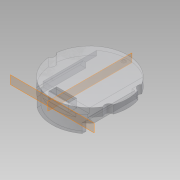
# Autodesk Inventor part: bottom2_2
Saved by Autodesk Inventor 2015 SP2 (Build 190223200, 223)
## iProperties
Created: 2015-01-05
Part Number: bottom2_2
Material: Acrylic
Document SubType Name: Modeling
Designer: Mathieu
Density: 1.188 g/cm^3
Appearance: Transparent - Clear
Mass: 1.09009 g
Surface Area: 15.2102 cm^2
Volume: 0.917582 cm^3
Author: Mathieu
Autodesk Inventor part; units mm, degrees
ref_plane "YZ Plane" through (0, 0, 0) normal (1, 0, 0) x (0, 1, 0)
ref_plane "XZ Plane" through (0, 0, 0) normal (0, 1, 0) x (-1, 0, 0)
ref_plane "XY Plane" through (0, 0, 0) normal (0, 0, 1) x (1, 0, 0)
sketch "Sketch10" plane through (0, 0, 0) normal (0, 1, 0) x (-1, 0, 0)
  circle A0 centre (0, 0) radius 12.25
  dimension "d115" = 24.5
  constraints: 1 centre point
  measures "d115" diameter of A0
extrude "Extrusion8" add sketch "Sketch10" along normal blind 2.7
sketch "Sketch15" plane through (0, 0, 0) normal (0, -1, 0) x (1, 0, 0)
  circle A0 centre (0, 0) radius 12.75 construction
  line L0 (12.75, 0) -> (0, 0) construction
  line L1 (0, 0) -> (-11.5554, -5.3884) construction
  line L2 (0, 0) -> (-11.5554, 5.3884) construction
  circle A1 centre (-11.5554, -5.3884) radius 1.375
  circle A2 centre (12.75, 0) radius 1.375
  circle A3 centre (-11.5554, 5.3884) radius 1.375
  dimension "d116" = 25.5
  dimension "d117" = 25
  dimension "d118" = 25
  dimension "d119" = 2.75
  constraints: 6 end point, 4 centre point, 4 coincident, 3 point on circle, 2 equal radius, 1 horizontal
  measures "d116" diameter of A0
  measures "d117" angle of L2 L0
  measures "d118" angle of L1 L0
  measures "d119" diameter of A2
extrude "Extrusion13" cut sketch "Sketch15" against normal up to surface (2.7 mm away)
sketch "Sketch17" plane through (0, 2.7, 0) normal (0, 1, 0) x (1, 0, 0)
  line L0 (-3.885, 10.76) -> (2.615, 10.76)
  line L1 (2.615, 10.76) -> (2.615, 8.16)
  line L2 (2.615, 8.16) -> (-3.885, 8.16)
  line L3 (-3.885, 8.16) -> (-3.885, 10.76)
  line L4 (2.615, 8.16) -> (-3.885, 10.76) construction
  line L5 (-3.885, 8.16) -> (2.615, 10.76) construction
  point P0 (0, 0)
  point P1 (-0.635, 9.46)
  dimension "d130" = 2.6
  dimension "d131" = 6.5
  dimension "d144" = 9.46
  dimension "d145" = 0.635
  constraints: 12 end point, 2 midpoint, 2 parallel, 1 horizontal, 1 perpendicular
  measures "d130" distance of L2.end L0.start
  measures "d131" distance of L1.end L2.end
  measures "d144" vertical distance of point (0, 0) point (-0.635, 9.46)
  measures "d145" horizontal distance of point (0, 0) point (-0.635, 9.46)
extrude "Extrusion14" cut sketch "Sketch17" against normal up to next
sketch "Sketch11" plane through (0, 0, 0) normal (0, -1, 0) x (1, 0, 0)
  line L0 (7.5, -7.7326) -> (-7.5, -7.7326)
  line L1 (-7.5, -7.7326) -> (-7.5, 12.25)
  line L2 (-7.5, 12.25) -> (7.5, 12.25)
  line L3 (7.5, 12.25) -> (7.5, -7.7326)
  arc A0 (12.1857, 1.2539) -> (12.1857, -1.2539) centre (12.75, 0) ccw projected
  arc A1 (-10.5141, -6.2863) -> (12.1857, -1.2539) centre (0, 0) ccw projected
  arc A2 (-10.5141, -6.2863) -> (-11.5739, -4.0135) centre (-11.5554, -5.3884) ccw projected
  arc A3 (-11.5739, 4.0135) -> (-11.5739, -4.0135) centre (0, 0) ccw projected
  arc A4 (-11.5739, 4.0135) -> (-10.5141, 6.2863) centre (-11.5554, 5.3884) ccw projected
  arc A5 (12.1857, 1.2539) -> (-10.5141, 6.2863) centre (0, 0) ccw projected
  dimension "d78" = 15
  dimension "d122" = 7.5
  constraints: 8 end point, 2 parallel, 1 horizontal, 1 perpendicular, 1 tangent
  measures "d78" distance of L0.start L0.end
  measures "d122" distance from line of point (0, 0) L3
extrude "Extrusion9" cut sketch "Sketch11" against normal blind 1.54 contours L0 L1 A5 L3 | A5 L2 L3 | L1 L2 A5
ref_plane "Work Plane4" through (0, 0, -12.25) normal (0, 0, -1) x (-1, 0, 0)
ref_plane "Work Plane3" through (0, 0, -7.7326) normal (-1, 0, 0) x (0, 0, 1)
sketch "Sketch13" plane through (0, 0, -12.25) normal (0, 0, -1) x (-1, 0, 0)
  line L0 (-7.5, 1.54) -> (-7.5, 0) projected
  line L1 (-12.1857, 0) -> (-7.5, 0) projected
  line L2 (-12.1857, 0) -> (-12.1857, 2.7) projected
  line L3 (10.5141, 2.7) -> (-12.1857, 2.7) projected
  line L4 (10.5141, 2.7) -> (10.5141, 0) projected
  line L5 (7.5, 0) -> (10.5141, 0) projected
  line L6 (7.5, 0) -> (7.5, 1.54) projected
  line L7 (7.5, 1.54) -> (-7.5, 1.54) projected
  line L8 (7.5, 0) -> (7.5, -1.6588)
  line L9 (7.5, -1.6588) -> (9.3, -1.6588)
  line L10 (9.3, -1.6588) -> (8.4, -0.1)
  line L11 (8.4, -0.1) -> (8.4, 0)
  line L12 (7.5, 0) -> (8.4, 0)
  line L13 (7.5, 0) -> (10.5141, 0) projected
  point P0 (0, 15)
  dimension "d146" = 0.9
  dimension "d147" = 60
  dimension "d148" = 1.8
  dimension "d149" = 0.1
  constraints: 10 end point, 2 perpendicular, 1 collinear, 1 point on line, 1 vertical
  measures "d146" distance between parallel lines of L8 L11
  measures "d147" angle of L9 L10
  measures "d148" distance of L8.end L9.end
  measures "d149" distance of L10.end L11.end
extrude "Extrusion11" add sketch "Sketch13" against normal blind 18.4 contours L5 L11 L10 L9 L8
mirror "Mirror1" about plane through (0, 0, -7.7326) normal (-1, 0, 0) of "Extrusion11"
sketch "Sketch14" plane through (0, 0, 0) normal (0, -1, 0) x (1, 0, 0)
  circle A0 centre (0, 0) radius 12.25
  arc A1 (7.5, 9.6857) -> (-7.5, 9.6857) centre (0, 0) ccw projected
  circle A2 centre (0, 0) radius 24.8523
  point P0 (1.5155, -12.4)
  constraints: 2 centre point, 2 coincident, 1 concentric
extrude "Extrusion12" cut sketch "Sketch14" along normal up to next
sketch "Sketch19" plane through (0, 0, 0) normal (0, -1, 0) x (1, 0, 0)
  arc A0 (-7.5, -8.3853) -> (7.5, -8.3853) centre (0, 0) ccw
  arc A1 (-7.5, -9.6857) -> (7.5, -9.6857) centre (0, 0) ccw projected
  line L0 (-7.5, -9.6857) -> (-7.5, 6.15) projected
  line L1 (7.5, -9.6857) -> (7.5, 6.15) projected
  point P0 (-7.5, -9.8747)
  point P1 (7.5, -9.8747)
  point P2 (-7.5, -9.7488)
  point P3 (7.5, -9.7488)
  dimension "d141" = 1
  constraints: 2 point on circle, 2 point on line, 1 centre point, 1 coincident, 1 other
extrude "Extrusion15" add sketch "Sketch19" along normal up to surface (1.6588 mm away)
sketch "Sketch21" plane through (0, 1.54, 0) normal (0, -1, 0) x (1, 0, 0)
  circle A0 centre (0, 11) radius 0.5
  point P0 (0, 0)
  dimension "d154" = 11
  dimension "d155" = 1
  constraints: 1 centre point, 1 vertical alignment
  measures "d154" distance of point (0, 0) A0.centre
  measures "d155" diameter of A0
extrude "Extrusion17" cut sketch "Sketch21" against normal blind 0.25
fillet "Fillet1" radius 0.25 2 edges at (-0.5, 1.79, 11) (-0.5, 1.54, 11)
sketch "Sketch22" plane through (0, -1.6588, 0) normal (0, -1, 0) x (1, 0, 0)
  arc A0 (-7.3, -9.8373) -> (7.3, -9.8373) centre (0, 0) ccw
  arc A1 (-7.3, -8.5599) -> (7.3, -8.5599) centre (0, 0) ccw
  line L0 (-7.3, -8.5599) -> (-7.3, -9.8373)
  line L1 (7.3, -8.5599) -> (7.3, -9.8373)
  arc A2 (-9.3, -7.9732) -> (-7.5, -9.6857) centre (0, 0) ccw projected
  arc A3 (-7.5, -9.6857) -> (7.5, -9.6857) centre (0, 0) ccw projected
  arc A4 (7.5, -9.6857) -> (9.3, -7.9732) centre (0, 0) ccw projected
  line L2 (9.3, -7.9732) -> (9.3, 6.15) projected
  line L3 (9.3, 6.15) -> (7.5, 6.15) projected
  line L4 (7.5, -8.3853) -> (7.5, 6.15) projected
  arc A5 (-7.5, -8.3853) -> (7.5, -8.3853) centre (0, 0) ccw projected
  line L5 (-7.5, -8.3853) -> (-7.5, 6.15) projected
  line L6 (-9.3, 6.15) -> (-7.5, 6.15) projected
  line L7 (-9.3, -7.9732) -> (-9.3, 6.15) projected
  arc A6 (-7.5, -8.3853) -> (7.5, -8.3853) centre (0, 0) ccw projected
  arc A7 (7.5, -9.6857) -> (9.3, -7.9732) centre (0, 0) ccw projected
  dimension "d163" = 0.2
  dimension "d164" = 0.2
  constraints: 4 end point, 4 point on circle, 2 centre point, 2 coincident, 2 concentric, 2 vertical
  measures "d163" distance between parallel lines of L5 L0
  measures "d164" distance between parallel lines of L1 L4
extrude "Extrusion18" add sketch "Sketch22" along normal blind 3.018 contours L0 A1 L1 A0
sketch "Sketch23" plane through (0, 0, 0) normal (0, -1, 0) x (1, 0, 0)
  arc A0 (-7.3, -8.5599) -> (7.3, -8.5599) centre (0, 0) ccw projected
  line L0 (-5.3558, -9.8933) -> (5.3558, -9.8933)
  line L1 (2.615, -10.76) -> (-3.284, -10.76) projected
  line L2 (-3.885, -8.16) -> (2.615, -8.16) projected
  dimension "d165" = 0.8667
  dimension "d166" = 2.6
  constraints: 2 end point, 2 point on circle, 1 horizontal
  measures "d165" distance between parallel lines of L1 L0
  measures "d166" distance between parallel lines of L1 L2
extrude "Extrusion19" add sketch "Sketch23" along normal blind 1
body "Solid2"
